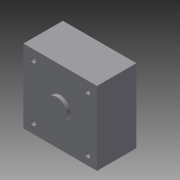
# Autodesk Inventor part: Motor
Saved by Autodesk Inventor 2015 (Build 190159000, 159)
## iProperties
Created: 2016-05-09
Part Number: Motor
Material: Generic
Document SubType Name: Modeling
Designer: Andreas
Density: 1 g/cm^3
Appearance: Default
Author: Andreas
Autodesk Inventor part; units mm, degrees
ref_plane "YZ Plane" through (0, 0, 0) normal (1, 0, 0) x (0, 1, 0)
ref_plane "XZ Plane" through (0, 0, 0) normal (0, 1, 0) x (-1, 0, 0)
ref_plane "XY Plane" through (0, 0, 0) normal (0, 0, 1) x (1, 0, 0)
sketch "Sketch1" plane through (0, 0, 0) normal (0, 1, 0) x (-1, 0, 0)
  line L0 (0, 0) -> (42, 0)
  line L1 (42, 0) -> (42, -42)
  line L2 (42, -42) -> (0, -42)
  line L3 (0, -42) -> (0, 0)
  dimension "d0" = 42
  dimension "d1" = 42
  constraints: 8 end point, 3 perpendicular, 1 horizontal
  measures "d0" distance of L0.start L0.end
  measures "d1" distance of L0.end L1.end
extrude "Extrusion1" add sketch "Sketch1" along normal blind 22.5
sketch "Sketch2" plane through (0, 22.5, 0) normal (0, 1, 0) x (1, 0, 0)
  circle A0 centre (-21, 21) radius 6
  line L0 (-42, 42) -> (-42, 0) projected
  line L1 (-42, 0) -> (0, 0) projected
  point P0 (-42, 21)
  point P1 (-21, 0)
  dimension "d4" = 12
  constraints: 2 midpoint, 1 centre point, 1 horizontal alignment, 1 vertical alignment
  measures "d4" diameter of A0
extrude "Extrusion2" add sketch "Sketch2" along normal blind 2 and the other way blind 24.5
sketch "Sketch3" plane through (-21, 24.5, -21) normal (0, 1, 0) x (1, 0, 0)
  circle A0 centre (0, 0) radius 2
  point P0 (21, -21)
  dimension "d7" = 4
  constraints: 1 centre point
  measures "d7" diameter of A0
extrude "Extrusion3" add sketch "Sketch3" along normal blind 11.5
sketch "Sketch4" plane through (0, 22.5, 0) normal (0, 1, 0) x (1, 0, 0)
  circle A0 centre (-5.5, 5.5) radius 1.5
  circle A1 centre (-36.4981, 5.5) radius 1.5
  circle A2 centre (-36.4981, 36.5) radius 1.5
  circle A3 centre (-5.5, 36.8446) radius 1.5
  line L0 (0, 0) -> (0, 42) projected
  line L1 (0, 42) -> (-42, 42) projected
  dimension "d10" = 3
  dimension "d11" = 3
  dimension "d12" = 3
  dimension "d13" = 3
  dimension "d14" = 31
  dimension "d15" = 31
  dimension "d16" = 5.5
  dimension "d17" = 5.5
  constraints: 4 centre point, 2 vertical alignment, 1 horizontal alignment
  measures "d10" diameter of A0
  measures "d11" diameter of A1
  measures "d12" diameter of A2
  measures "d13" diameter of A3
  measures "d14" distance of A3.centre A2.centre
  measures "d15" distance of A1.centre A2.centre
  measures "d16" distance from line of L0 A3.centre
  measures "d17" distance from line of L1 A2.centre
extrude "Extrusion4" cut sketch "Sketch4" against normal up to next
body "Solid1"
